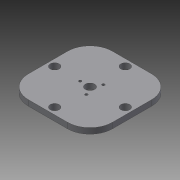
# Autodesk Inventor part: Vertical_Lead_Screw_Plate
Saved by Autodesk Inventor 2015 (Build 190159000, 159)
## iProperties
Created: 2014-12-22
Part Number: Vertical_Lead_Screw_Plate
Material: Generic
Document SubType Name: Modeling
Designer: Drew
Density: 1 g/cm^3
Appearance: Default
Author: Drew
Autodesk Inventor part; units mm, degrees
ref_plane "YZ Plane" through (0, 0, 0) normal (1, 0, 0) x (0, 1, 0)
ref_plane "XZ Plane" through (0, 0, 0) normal (0, 1, 0) x (-1, 0, 0)
ref_plane "XY Plane" through (0, 0, 0) normal (0, 0, 1) x (1, 0, 0)
sketch "Sketch3" plane through (0, 0, 0) normal (0, 1, 0) x (-1, 0, 0)
  circle A0 centre (11.1125, 0) radius 1.4906
  circle A1 centre (-5.5563, 9.6237) radius 1.4906
  circle A2 centre (-5.5562, -9.6237) radius 1.4906
  circle A3 centre (0, 0) radius 5.25
  line L0 (0, 0) -> (11.1125, 0)
  line L1 (0, 0) -> (-5.5563, 9.6237)
  line L2 (0, 0) -> (-5.5562, -9.6237)
  line L3 (0, 11.7306) -> (0, -34.9786)
  line L4 (38.6398, 0) -> (-3.2951, 0)
  circle A4 centre (40, 0) radius 5.05
  circle A5 centre (0, -40) radius 5.05
  circle A6 centre (0, 40) radius 5.05
  circle A7 centre (-40, 0) radius 5.05
  line L5 (-47.625, -47.625) -> (47.625, -47.625)
  line L6 (47.625, -47.625) -> (47.625, 47.625)
  line L7 (47.625, 47.625) -> (-47.625, 47.625)
  line L8 (-47.625, 47.625) -> (-47.625, -47.625)
  line L9 (-47.625, -47.625) -> (47.625, 47.625) construction
  line L10 (47.625, -47.625) -> (-47.625, 47.625) construction
  dimension "d19" = 120
  dimension "d20" = 120
  dimension "d21" = 11.1125
  dimension "d22" = 11.1125
  dimension "d23" = 11.1125
  dimension "d24" = 2.9811
  dimension "d25" = 2.9811
  dimension "d26" = 2.9811
  dimension "d27" = 80
  dimension "d28" = 80
  dimension "d29" = 10.1
  dimension "d30" = 10.1
  dimension "d31" = 95.25
  dimension "d32" = 95.25
  dimension "d36" = 10.5
  constraints: 22 end point, 8 centre point, 4 midpoint, 4 point on line, 3 horizontal, 2 parallel, 2 symmetric about line, 1 perpendicular, 1 vertical, 4 other
  measures "d19" angle of L1 L0
  measures "d20" angle of L0 L2
  measures "d21" distance of L0.end point (0, 0)
  measures "d22" distance of L2.start L2.end
  measures "d23" distance of L0.start L1.end
  measures "d24" diameter of A0
  measures "d25" diameter of A1
  measures "d26" diameter of A2
  measures "d27" diameter of A4.centre L3
  measures "d28" diameter of A5.centre L0
  measures "d29" diameter of A4
  measures "d30" diameter of A5
  measures "d31" distance of L5.end L6.end
  measures "d32" distance of L6.end L7.end
  measures "d36" diameter of A3
extrude "Extrusion6" add sketch "Sketch3" along normal blind 6.35
fillet "Fillet1" radius 25.4 4 edges at (-47.625, 3.175, 47.625) (47.625, 3.175, 47.625) (47.625, 3.175, -47.625) (-47.625, 3.175, -47.625)
equation "\"d22\" = d21"
equation "\"d23\" = d21"
equation "\"d25\" = d24"
equation "\"d26\" = d24"
equation "\"d28\" = d27"
equation "\"d30\" = d29"
equation "\"d32\" = d31"
body "Solid5"
